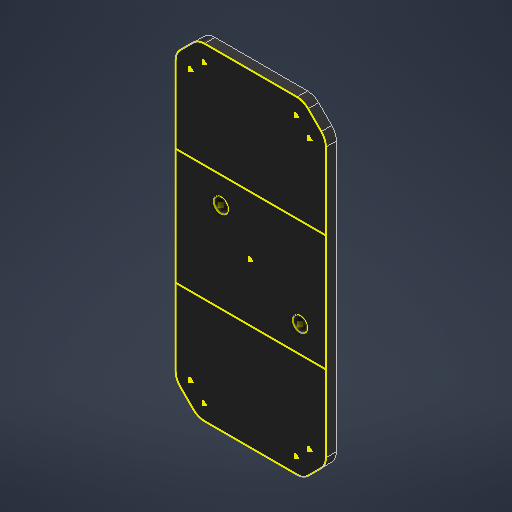
# Autodesk Inventor part: Solenoid Board
Saved by Autodesk Inventor 2026.1 (Build 301233020, 233B)
## iProperties
Created: 2025-11-08
Part Number: Solenoid Board
Material: Generic
Document SubType Name: Modeling
Designer: Bahaa
Density: 1 g/cm^3
Appearance: Default
Mass: 3.436 g
Surface Area: 38.0998 cm^2
Volume: 3.436 cm^3
Author: Bahaa
Autodesk Inventor part; units mm, degrees
ref_plane "YZ Plane" through (0, 0, 0) normal (1, 0, 0) x (0, 1, 0)
ref_plane "XZ Plane" through (0, 0, 0) normal (0, 1, 0) x (-1, 0, 0)
ref_plane "XY Plane" through (0, 0, 0) normal (0, 0, 1) x (1, 0, 0)
sketch "Sketch1" plane through (0, 0, 0) normal (0, 1, 0) x (-1, 0, 0)
  line L0 (14.25, 11) -> (-14.25, 11)
  line L1 (-14.25, 11) -> (-14.25, -11)
  line L2 (-14.25, -11) -> (14.25, -11)
  line L3 (14.25, -11) -> (14.25, 11)
  line L4 (14.25, 11) -> (-14.25, -11) construction
  line L5 (-14.25, 11) -> (14.25, -11) construction
  line L6 (14.25, 11) -> (5.65, 11)
  line L7 (5.65, 11) -> (5.65, 6) construction
  line L8 (5.65, 6) -> (14.25, 6) construction
  line L9 (14.25, 6) -> (14.25, 11)
  line L10 (-14.25, -11) -> (-9.35, -11)
  line L11 (-9.35, -11) -> (-9.35, -6) construction
  line L12 (-14.25, -6) -> (-14.25, -11)
  circle A0 centre (5.65, 6) radius 1.35
  circle A1 centre (-9.35, -6) radius 1.35
  line L13 (10.0074, 31) -> (14.25, 26.7574)
  line L14 (10.0074, 31) -> (-10.0074, 31)
  line L15 (-14.25, 26.7574) -> (-14.25, 11)
  line L16 (14.25, 0) -> (-14.25, 0) construction
  line L17 (14.25, -26.7574) -> (14.25, 4.1382)
  line L18 (10.0074, -31) -> (14.25, -26.7574)
  line L19 (10.0074, -31) -> (-10.0074, -31)
  line L20 (-14.25, -26.7574) -> (-14.25, -11)
  line L21 (14.25, 11) -> (14.25, 26.7574)
  line L22 (-10.0074, 31) -> (-14.25, 26.7574)
  line L23 (-14.25, -26.7574) -> (-10.0074, -31)
  point P0 (0, 0)
  point P1 (-14.25, 31)
  point P2 (-14.25, -31)
  point P3 (14.25, -11)
  point P4 (0, 0)
  dimension "d0" = 28.5
  dimension "d1" = 22
  dimension "d2" = 8.6
  dimension "d3" = 5
  dimension "d5" = 5
  dimension "d6" = 2.7
  dimension "d7" = 2.7
  dimension "d22" = 23.6
  dimension "d23" = 135
  dimension "d25" = 6
  dimension "d27" = 135
  dimension "d39" = 20
  dimension "d44" = 6
  dimension "d45" = 135
  dimension "d48" = 135
  dimension "d49" = 6
  constraints: 48 end point, 5 midpoint, 5 parallel, 4 horizontal, 4 point on line, 3 perpendicular, 3 symmetric about line, 2 centre point, 2 coincident, 2 collinear
  measures "d0" distance of L2.end L1.end
  measures "d1" distance of L2.end L0.start
  measures "d2" distance of L8.end L7.end
  measures "d3" distance of L7.end L6.end
  measures "d5" distance of L11.end L10.end
  measures "d6" diameter of A0
  measures "d7" diameter of A1
  measures "d22" distance from line of L3 L11.end
  measures "d23" angle of L13 L21
  measures "d25" distance of L13.start L13.end
  measures "d27" angle of L18 L17
  measures "d39" distance of point (-14.25, 31) L0.end
  measures "d44" distance of L14.end L15.start
  measures "d45" angle of L15 L22
  measures "d48" angle of L20 L23
  measures "d49" distance of L20.start L19.end
extrude "Extrusion1" add sketch "Sketch1" along normal blind 2
fillet "Fillet1" radius 3 8 edges at (-10.0074, 1, 31) (-14.25, 1, 26.7574) (-14.25, 1, -26.7574) (-10.0074, 1, -31) (10.0074, 1, 31) (14.25, 1, 26.7574) (10.0074, 1, -31) (14.25, 1, -26.7574)
fillet "Fillet2" [suppressed]
extrude "Extrusion2" [suppressed]
fillet "Fillet3" [suppressed]
sketch "Sketch2" plane through (0, 0, 0) normal (0, -1, 0) x (1, 0, 0)
  line L0 (14.25, -11) -> (-14.25, -11) projected
  line L1 (-14.25, 11) -> (14.25, 11) projected
  arc A0 (13.3713, -27.636) -> (14.25, -25.5147) centre (11.25, -25.5147) ccw projected
  line L2 (14.25, 25.5147) -> (14.25, -25.5147) projected
  arc A1 (14.25, 25.5147) -> (13.3713, 27.636) centre (11.25, 25.5147) ccw projected
  line L3 (10.886, 30.1213) -> (13.3713, 27.636) projected
  arc A2 (10.886, 30.1213) -> (8.7647, 31) centre (8.7647, 28) ccw projected
  line L4 (-8.7647, 31) -> (8.7647, 31) projected
  arc A3 (-8.7647, 31) -> (-10.886, 30.1213) centre (-8.7647, 28) ccw projected
  line L5 (-13.3713, 27.636) -> (-10.886, 30.1213) projected
  arc A4 (-13.3713, 27.636) -> (-14.25, 25.5147) centre (-11.25, 25.5147) ccw projected
  line L6 (-14.25, -25.5147) -> (-14.25, 25.5147) projected
  arc A5 (-14.25, -25.5147) -> (-13.3713, -27.636) centre (-11.25, -25.5147) ccw projected
  line L7 (-10.886, -30.1213) -> (-13.3713, -27.636) projected
  arc A6 (-10.886, -30.1213) -> (-8.7647, -31) centre (-8.7647, -28) ccw projected
  line L8 (8.7647, -31) -> (-8.7647, -31) projected
  arc A7 (8.7647, -31) -> (10.886, -30.1213) centre (8.7647, -28) ccw projected
  line L9 (13.3713, -27.636) -> (10.886, -30.1213) projected
  circle A8 centre (-5.65, 6) radius 1.35 projected
  circle A9 centre (9.35, -6) radius 1.35 projected
  point P0 (0, 0)
equation "\"d27\" = d23"
body "Solid1"
